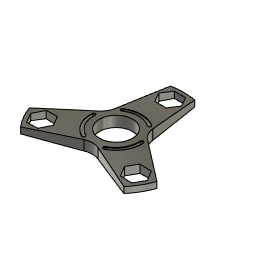
Final Fidget Spinner v1 (Autodesk Fusion 360 design; units mm, degrees)
Autodesk Fusion 360 part; units mm, degrees
sketch "Sketch1" plane through (0, 0, 0) normal (0, 0, 1) x (1, 0, 0)
  circle A0 centre (0, 0) radius 45
  circle A1 centre (0, 0) radius 11
  circle A2 centre (0, 0) radius 4
  circle A3 centre (0, 0) radius 13.5
  line L0 (7.5056, 36) -> (3.7528, 42.5)
  line L1 (3.7528, 42.5) -> (-3.7528, 42.5)
  line L2 (-3.7528, 42.5) -> (-7.5056, 36)
  line L3 (-7.5056, 36) -> (-3.7528, 29.5)
  line L4 (-3.7528, 29.5) -> (3.7528, 29.5)
  line L5 (3.7528, 29.5) -> (7.5056, 36)
  line L6 (0, 0) -> (0, 29.5) construction
  circle A4 centre (0, 36) radius 9 construction
  line L7 (-13.3941, 1.6875) -> (-8.0282, 44.2781)
  line L8 (8.0282, 44.2781) -> (13.3941, 1.6875)
  point P0 (0, 36)
  dimension "d1" = 90
  dimension "d2" = 22
  dimension "d3" = 8
  dimension "d4" = 2.5
  dimension "d5" = 6.5
  dimension "d6" = 29.5
  constraint coincident A0.centre A1.centre
  constraint concentric A1 A2
  constraint midpoint L4 L6.end
  constraint vertical L6
  constraint perpendicular L4 L6
  constraint coincident P0 A4.centre
  constraint tangent A0 A4
  constraint coincident A3 L7.start
  constraint coincident A0 L7.end
  constraint tangent A3 L7
  constraint tangent A4 L7
  constraint coincident A0 L8.start
  constraint coincident A3 L8.end
  constraint tangent A3 L8
  constraint tangent A4 L8
  measures "d1" diameter of A0
  measures "d2" diameter of A1
  measures "d3" diameter of A2
  measures "d4" distance of A1 A3
  measures "d5" distance of P0 L5
  measures "d6" distance of A0.centre L6.end
extrude "Extrude1" add sketch "Sketch1" along normal blind 8 contours A0 A3 L7 L8 | A3 picked at (0, 24.1667) makes body 1
sketch "Sketch3" plane through (0, 0, 8) normal (0, 0, 1) x (-1, 0, 0)
  circle A0 centre (0, 0) radius 11
  line L0 (-7.5056, -36) -> (-3.7528, -29.5)
  line L1 (-3.7528, -29.5) -> (3.7528, -29.5)
  line L2 (3.7528, -29.5) -> (7.5056, -36)
  line L3 (7.5056, -36) -> (3.7528, -42.5)
  line L4 (3.7528, -42.5) -> (-3.7528, -42.5)
  line L5 (-3.7528, -42.5) -> (-7.5056, -36)
  arc A1 (13.3941, -1.6875) -> (-13.3941, -1.6875) centre (0, 0) ccw
  line L6 (-13.3941, -1.6875) -> (-8.0282, -44.2781)
  arc A2 (-8.0282, -44.2781) -> (8.0282, -44.2781) centre (0, 0) ccw
  line L7 (8.0282, -44.2781) -> (13.3941, -1.6875)
  line L8 (9, -13.2288) -> (-9, -13.2288) construction
  arc A3 (-9.5625, -14.0556) -> (9.5625, -14.0556) centre (0, 0) ccw
  arc A4 (-8.4375, -12.402) -> (8.4375, -12.402) centre (0, 0) ccw
  arc A5 (9.5625, -14.0556) -> (8.4375, -12.402) centre (9, -13.2288) ccw
  arc A6 (-8.4375, -12.402) -> (-9.5625, -14.0556) centre (-9, -13.2288) ccw
  dimension "d17" = 30
  dimension "d18" = 34
  dimension "d19" = 18
  constraint coincident A0.centre A1.centre
  constraint concentric A3 A4
  constraint tangent A3 A5
  constraint tangent A4 A5
  constraint tangent A3 A6
  constraint tangent A4 A6
  constraint coincident L8.start A5.centre
  constraint coincident L8.end A6.centre
  constraint horizontal L8
  measures "d17" diameter of A4
  measures "d18" diameter of A3
  measures "d19" distance of L8.start L8.end
extrude "Extrude3" cut sketch "Sketch3" against normal blind 2 contours A3 A4 A5 A6 bodies 1
sketch "Sketch4" plane through (0, 0, 0) normal (0, 0, -1) x (1, 0, 0)
  circle A0 centre (0, 0) radius 11
  line L0 (3.7528, -29.5) -> (7.5056, -36)
  line L1 (7.5056, -36) -> (3.7528, -42.5)
  line L2 (3.7528, -42.5) -> (-3.7528, -42.5)
  line L3 (-3.7528, -42.5) -> (-7.5056, -36)
  line L4 (-7.5056, -36) -> (-3.7528, -29.5)
  line L5 (-3.7528, -29.5) -> (3.7528, -29.5)
  arc A1 (13.3941, -1.6875) -> (-13.3941, -1.6875) centre (0, 0) ccw
  line L6 (-13.3941, -1.6875) -> (-8.0282, -44.2781)
  arc A2 (-8.0282, -44.2781) -> (8.0282, -44.2781) centre (0, 0) ccw
  line L7 (8.0282, -44.2781) -> (13.3941, -1.6875)
  line L8 (9, -13.2288) -> (-9, -13.2288) construction
  arc A3 (-9.5625, -14.0556) -> (9.5625, -14.0556) centre (0, 0) ccw
  arc A4 (-8.4375, -12.402) -> (8.4375, -12.402) centre (0, 0) ccw
  arc A5 (-8.4375, -12.402) -> (-9.5625, -14.0556) centre (-9, -13.2288) ccw
  arc A6 (9.5625, -14.0556) -> (8.4375, -12.402) centre (9, -13.2288) ccw
  dimension "d22" = 30
  dimension "d23" = 34
  dimension "d24" = 18
  constraint coincident A0.centre A1.centre
  constraint concentric A0 A3
  constraint tangent A4 A6
  constraint tangent A4 A5
  constraint tangent A3 A6
  constraint tangent A3 A5
  constraint coincident L8.start A6.centre
  constraint coincident L8.end A5.centre
  constraint horizontal L8
  measures "d22" diameter of A4
  measures "d23" diameter of A3
  measures "d24" distance of L8.start L8.end
extrude "Extrude4" cut sketch "Sketch4" against normal blind 2 contours A3 A4 A5 A6 bodies 1
fillet "Fillet2" radius 1 8 edges at (0, 17, 2) (-9.8268, 12.6663, 2) (0, 15, 2) (9.8268, 12.6663, 2) (0, 15, 6) (-9.8268, 12.6663, 6) (0, 17, 6) (9.8268, 12.6663, 6) on bodies 1
sketch "Sketch2" plane through (0, 0, 0) normal (1, 0, 0) x (0, 1, 0)
  line L0 (0.0041, 8.0893) -> (45, 6)
  line L1 (0, 0) -> (45, 2)
  line L2 (45, 8) -> (44.2781, 8)
  line L3 (45, 0) -> (44.2781, 0)
  line L4 (0.0041, 8.0893) -> (45, 8)
  line L5 (0, 0) -> (45, 0)
  line L6 (45, 6) -> (45, 8)
  line L7 (45, 0) -> (45, 2)
  dimension "d13" = 2
  dimension "d14" = 2
  constraint coincident L1.start L5.start
  constraint coincident L2.start L4.end
  constraint coincident L3.start L5.end
  constraint coincident L2 L4.end
  constraint coincident L4 L2.start
  constraint vertical L6
  constraint vertical L7
  constraint equal L0 L1
  measures "d13" distance of L0.end L2
  measures "d14" distance of L1.end L3
revolve "Revolve1" cut sketch "Sketch2" angle 360 about axis through (0, 0, 1.75) along (0, 0, 1) bodies 1
pattern_circular "C-Pattern3" count 3 over 360 about axis through (0, 0, 1.75) along (0, 0, 1) of bodies 1 makes body 2 at (-18.3581, -13.7962, 7.0232) makes body 3 at (21.1269, -9.0005, 7.0232)
combine "Combine3" operation add target body 3 tool bodies 2 1
fillet "Fillet4" radius 12 3 edges at (0, -14.6463, 4.0302) (12.6841, 7.3232, 4.0302) (-12.6841, 7.3232, 4.0302) on bodies 3
